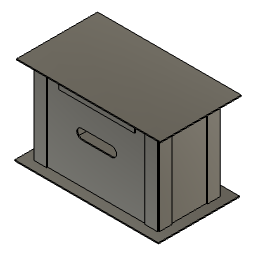
Part1, 3D Box (Autodesk Fusion 360 design; units mm, degrees)
Autodesk Fusion 360 part; units mm, degrees
sketch "Sketch1" plane through (0, 0, 0) normal (0, 1, 0) x (1, 0, 0)
  line L0 (0, 0) -> (304.8, 0)
  line L1 (304.8, 0) -> (304.8, -203.2)
  line L2 (304.8, -203.2) -> (0, -203.2)
  line L3 (0, -203.2) -> (0, 0)
  line L4 (152.4, -203.2) -> (152.4, -171.45) construction
  line L5 (152.4, -203.2) -> (152.4, -114.3) construction
  line L6 (114.9, -126.8) -> (189.9, -126.8)
  arc A0 (189.9, -126.8) -> (189.9, -101.8) centre (189.9, -114.3) ccw
  line L7 (189.9, -101.8) -> (114.9, -101.8)
  arc A1 (114.9, -101.8) -> (114.9, -126.8) centre (114.9, -114.3) ccw
  line L8 (114.9, -114.3) -> (189.9, -114.3) construction
  point P0 (152.4, -114.3)
  dimension "d11" = 304.8
  dimension "d12" = 203.2
  dimension "d25" = 31.75
  dimension "d26" = 88.9
  dimension "d27" = 25
  constraint horizontal L0
  constraint vertical L1
  constraint horizontal L2
  constraint vertical L3
  constraint coincident L0.start L3.end
  constraint midpoint L2 L4.start
  constraint perpendicular L2 L4
  constraint perpendicular L2 L5
  constraint tangent L6 A0
  constraint tangent A0 L7
  constraint parallel L6 L7
  constraint tangent L7 A1
  constraint tangent L6 A1
  constraint perpendicular L5 L8
  constraint coincident P0 L5.end
  constraint midpoint L8 P0
  measures "d11" distance of L0.start L0.end
  measures "d12" distance of L0.start L2.end
  measures "d25" distance of L4.start L4.end
  measures "d26" distance of L4.start P0
  measures "d27" diameter of A0
extrude "Extrude2" add sketch "Sketch1" along normal blind 2.5 makes body 1
sketch "Sketch14" plane through (0, 0, 0) normal (1, 0, 0) x (0, 1, 0)
  line L0 (0, 0) -> (2.5, 0) construction
  line L1 (2.5, 0) -> (149.9, 0)
  line L2 (149.9, 0) -> (149.9, 203.2)
  line L3 (149.9, 203.2) -> (2.5, 203.2)
  line L4 (2.5, 203.2) -> (2.5, 0)
  dimension "d103" = 2.5
  dimension "d104" = 147.4
  dimension "d105" = 203.2
  constraint coincident L0.start origin
  constraint horizontal L0
  constraint horizontal L1
  constraint vertical L2
  constraint horizontal L3
  constraint vertical L4
  measures "d103" distance of L0.start L0.end
  measures "d104" distance of L0.end L1.end
  measures "d105" distance of L0.end L3.end
extrude "Extrude4" add sketch "Sketch1" against normal blind 2.5 from surface at 152.4 separate body contours L0 L1 L2 L3 | L6 A0 L7 A1 makes body 2
sketch "Sketch6" plane through (0, 0, 0) normal (0, 0, 1) x (1, 0, 0)
  line L0 (-50, 75) -> (375, 75) construction
  line L1 (150, 175) -> (150, -56.0201) construction
  line L2 (-27.9, -25.4) -> (332.7, -25.4)
  line L3 (332.7, -25.4) -> (332.7, 177.8)
  line L4 (332.7, 177.8) -> (-27.9, 177.8)
  line L5 (-27.9, 177.8) -> (-27.9, -25.4)
  line L6 (0, 0) -> (304.8, 0)
  line L7 (307.3, 0) -> (307.3, 152.4)
  line L8 (0, 0) -> (0, 152.4)
  line L9 (-2.5, 0) -> (-2.5, 152.4)
  line L10 (0, 152.4) -> (304.8, 152.4)
  dimension "d51" = 25.4
  dimension "d53" = 25.4
  dimension "d55" = 25.4
  dimension "d56" = 25.4
  constraint horizontal L0
  constraint vertical L1
  constraint horizontal L2
  constraint vertical L3
  constraint horizontal L4
  constraint vertical L5
  measures "d51" distance of L2 L6
  measures "d53" distance of L3 L7
  measures "d55" distance of L5 L9
  measures "d56" distance of L4 L10
extrude "Extrude5" add sketch "Sketch6" against normal blind 2.5 separate body makes body 3
sketch "Sketch7" plane through (307.3, 0, 0) normal (1, 0, 0) x (0, 1, 0)
  line L0 (0, 203.2) -> (0, 0)
  line L1 (0, 0) -> (152.4, 0)
  line L2 (152.4, 0) -> (152.4, 203.2)
  line L3 (152.4, 203.2) -> (0, 203.2)
  line L4 (0, 0) -> (31.75, 0)
  line L5 (31.75, 0) -> (31.75, 203.2)
  line L6 (31.75, 203.2) -> (0, 203.2)
  line L7 (0, 203.2) -> (0, 0)
  dimension "d59" = 31.75
  dimension "d60" = 203.2
  constraint horizontal L4
  constraint vertical L5
  constraint horizontal L6
  constraint vertical L7
  constraint coincident L0.end L1.start
  measures "d59" distance of L0.end L4.end
  measures "d60" distance of L0.end L0.start
sketch "Sketch12" plane through (0, 0, 0) normal (0, 1, 0) x (1, 0, 0)
  line L0 (304.8, 0) -> (307.3, 0) construction
  line L1 (307.3, 0) -> (275.55, 0)
  line L2 (275.55, 0) -> (275.55, -203.2)
  line L3 (275.55, -203.2) -> (307.3, -203.2)
  line L4 (307.3, -203.2) -> (307.3, 0)
  dimension "d69" = 2.5
  dimension "d70" = 203.2
  dimension "d71" = 31.75
  constraint horizontal L0
  constraint horizontal L1
  constraint vertical L2
  constraint horizontal L3
  constraint vertical L4
  measures "d69" distance of L0.start L0.end
  measures "d70" distance of L0.end L3.end
  measures "d71" distance of L2 L4
extrude "Extrude8" add sketch "Sketch12" against normal blind 2.5 separate body makes body 4
extrude "Extrude9" add sketch "Sketch7" along normal blind 2.5 contours L0 L1 L3 L4 L5 L6 L7 bodies 4
ref_plane "WorkPlane1" through (152.4, 76.2, 101.6) normal (1, 0, 0) x (0, 0, -1)
mirror "Mirror1" about plane through (152.4, 76.2, 101.6) normal (1, 0, 0) of bodies 4 makes body 5
ref_plane "WorkPlane2" through (152.4, 76.2, 101.6) normal (0, -1, 0) x (-1, 0, 0)
mirror "Mirror2" about plane through (152.4, 76.2, 101.6) normal (0, -1, 0) of bodies 5 makes body 6
mirror "Mirror3" about plane through (152.4, 76.2, 101.6) normal (1, 0, 0) of bodies 6 makes body 7
extrude "Extrude10" add 1 faces at (92.3, 110.0667, 0) along direction (0, 0, 1) blind 2.5 from surface at 205.7 separate body on bodies 3 makes body 8
move_body "Move4" bodies 8 to x (1, 0, 0) y (0, 1, 0) z (0, 0, 1) at (0, 0, -2.5)
sketch "Sketch13" plane through (0, 0, 205.7) normal (0, 0, 1) x (-1, 0, 0)
  line L0 (27.9, -177.8) -> (27.9, 25.4)
  line L1 (27.9, 25.4) -> (-332.7, 25.4)
  line L2 (-332.7, 25.4) -> (-332.7, -177.8)
  line L3 (-332.7, -177.8) -> (27.9, -177.8)
  line L4 (-152.4, 25.4) -> (-152.4, -177.8) construction
  line L5 (-152.4, -0.047) -> (-152.4, -2.547) construction
  line L6 (-152.4, -2.547) -> (-152.4, -5.047) construction
  line L7 (-247.65, -5.047) -> (-57.15, -5.047)
  line L8 (-57.15, -5.047) -> (-57.15, -2.547)
  line L9 (-57.15, -2.547) -> (-247.65, -2.547)
  line L10 (-247.65, -2.547) -> (-247.65, -5.047)
  line L11 (-247.65, -5.047) -> (-57.15, -2.547) construction
  line L12 (-57.15, -5.047) -> (-247.65, -2.547) construction
  line L13 (-152.4, -0.047) -> (-152.4, 2.453) construction
  line L14 (-152.4, 2.453) -> (-152.4, 4.953) construction
  line L15 (-247.65, 4.953) -> (-57.15, 4.953)
  line L16 (-57.15, 4.953) -> (-57.15, 2.453)
  line L17 (-57.15, 2.453) -> (-247.65, 2.453)
  line L18 (-247.65, 2.453) -> (-247.65, 4.953)
  line L19 (-247.65, 4.953) -> (-57.15, 2.453) construction
  line L20 (-57.15, 4.953) -> (-247.65, 2.453) construction
  point P0 (-152.4, -3.797)
  point P1 (-152.4, 3.703)
  dimension "d88" = 2.5
  dimension "d89" = 2.5
  dimension "d90" = 190.5
  dimension "d91" = 2.5
  dimension "d92" = 2.5
  dimension "d93" = 2.5
  dimension "d94" = 190.5
  dimension "d95" = 2.5
  constraint midpoint L1 L4.start
  constraint midpoint L3 L4.end
  constraint coincident L4 L5.start
  constraint parallel L4 L5
  constraint parallel L4 L6
  constraint horizontal L7
  constraint perpendicular L7 L8
  constraint parallel L7 L9
  constraint parallel L8 L10
  constraint coincident L11 P0
  constraint coincident L12 P0
  constraint midpoint L6 P0
  constraint parallel L4 L13
  constraint vertical L14
  constraint horizontal L15
  constraint perpendicular L15 L16
  constraint parallel L15 L17
  constraint parallel L16 L18
  constraint coincident L19 P1
  constraint coincident L20 P1
  constraint midpoint L14 P1
  measures "d88" distance of L5.start L5.end
  measures "d89" distance of L5.end L6.end
  measures "d90" distance of L8.end L9.end
  measures "d91" distance of L7.end L8.end
  measures "d92" distance of L5.start L13.end
  measures "d93" distance of L13.end L14.end
  measures "d94" distance of L16.end L17.end
  measures "d95" distance of L15.end L16.end
extrude "Extrude11" add sketch "Sketch13" along normal blind 31.75 separate body contours L7 L8 L9 L10 makes body 9
extrude "Extrude12" add sketch "Sketch13" along normal blind 31.75 separate body contours L15 L16 L17 L18 makes body 10
mirror "Mirror4" about plane through (152.4, 76.2, 101.6) normal (0, -1, 0) of bodies 9 10 makes body 11 at (120.65, 149.853, 216.2833) makes body 12 at (184.15, 157.353, 216.2833)
combine "Combine1" operation add target body 8 tool bodies 9 10 11 12
move_body "Move5" bodies 8 to x (-1, 0, 0) y (0, 1, 0) z (0, 0, -1) at (609.6, 0, 0)
move_body "Move6" bodies 8 to x (1, 0, 0) y (0, 1, 0) z (0, 0, 1) at (-300, 0, 450)
move_body "Move7" bodies 8 to x (1, 0, 0) y (0, 1, 0) z (0, 0, 1) at (0, 0, -25)
extrude "Extrude14" add sketch "Sketch14" along normal blind 2.5 from surface at 304.8 separate body makes body 13
sketch "Sketch15" plane through (0, 0, 0) normal (1, 0, 0) x (0, 1, 0)
  line L0 (0, 0) -> (2.5, 0) construction
  line L1 (2.5, 0) -> (152.4, 0)
  line L2 (152.4, 0) -> (152.4, 203.2)
  line L3 (152.4, 203.2) -> (2.5, 203.2)
  line L4 (2.5, 203.2) -> (2.5, 0)
  dimension "d111" = 2.5
  dimension "d112" = 149.9
  dimension "d113" = 203.2
  constraint coincident L0.start origin
  constraint horizontal L0
  constraint horizontal L1
  constraint vertical L2
  constraint horizontal L3
  constraint vertical L4
  measures "d111" distance of L0.start L0.end
  measures "d112" distance of L0.end L1.end
  measures "d113" distance of L0.end L3.end
extrude "Extrude15" add sketch "Sketch15" against normal blind 2.5 separate body makes body 14
equation "box_length = 304.8 mm" comment "12 inches"
equation "box_width = 152.4 mm" comment "6 inches"
equation "box_height = 203.2 mm" comment "8 inches"
equation "base_length = 342.9 mm" comment "13.5 inches"
equation "base_width = 190.5 mm" comment "7.5 inches"
equation "carboard_thickness = 2.5 mm"
equation "post_width = 31.75 mm" comment "1.25 inches"
equation "divit_length = 190.5 mm" comment "7.5 inches"
equation "hole_width = 25 mm"
equation "hole_length = 75 mm"
equation "d11 = box_length"
equation "d12 = box_height"
equation "divit_height = 31.75 mm" comment "1.25 inches"
equation "hole_center_from_top = 88.9 mm" comment "3.5  inches"
equation "d25 = divit_height"
equation "d26 = hole_center_from_top"
equation "d27 = hole_width"
equation "d30 = carboard_thickness"
equation "d45 = box_width"
equation "d46 = -carboard_thickness"
equation "base_extension = 25.4 mm" comment "1 inch"
equation "d51 = base_extension"
equation "d53 = base_extension"
equation "d55 = base_extension"
equation "d56 = base_extension"
equation "d57 = -carboard_thickness"
equation "d59 = post_width"
equation "d60 = box_height"
equation "d69 = carboard_thickness"
equation "d70 = box_height"
equation "d71 = post_width"
equation "d72 = carboard_thickness * -1"
equation "d74 = carboard_thickness"
equation "d82 = box_height + carboard_thickness"
equation "d83 = carboard_thickness"
equation "d87 = carboard_thickness * -1"
equation "d88 = carboard_thickness"
equation "d89 = carboard_thickness"
equation "d90 = divit_length"
equation "d91 = carboard_thickness"
equation "d92 = carboard_thickness"
equation "d93 = carboard_thickness"
equation "d94 = divit_length"
equation "d95 = carboard_thickness"
equation "d96 = divit_height"
equation "d98 = divit_height"
equation "d103 = carboard_thickness"
equation "d104 = box_width - 2 * carboard_thickness"
equation "d105 = box_height"
equation "d108 = box_length"
equation "d109 = carboard_thickness"
equation "d111 = carboard_thickness"
equation "d112 = box_width - carboard_thickness"
equation "d113 = box_height"
equation "d114 = carboard_thickness * -1"
